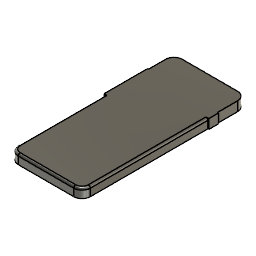
case (Autodesk Fusion 360 design; units mm, degrees)
Autodesk Fusion 360 part; units mm, degrees
sketch "Sketch1" plane through (0, 0, 0) normal (0, 0, 1) x (1, 0, 0)
  line L0 (28.485, 84.19) -> (0, 84.19)
  line L1 (36.985, 0) -> (36.985, 75.69)
  line L2 (0, 0) -> (0, 84.19) construction
  line L3 (0, 0) -> (36.985, 0) construction
  arc A0 (36.985, 75.69) -> (28.485, 84.19) centre (28.485, 75.69) ccw
  line L4 (-28.485, 84.19) -> (0, 84.19)
  arc A1 (-28.485, 84.19) -> (-36.985, 75.69) centre (-28.485, 75.69) ccw
  line L5 (-36.985, 0) -> (-36.985, 75.69)
  line L6 (36.985, 0) -> (36.985, -75.69)
  arc A2 (28.485, -84.19) -> (36.985, -75.69) centre (28.485, -75.69) ccw
  line L7 (28.485, -84.19) -> (0, -84.19)
  line L8 (-28.485, -84.19) -> (0, -84.19)
  arc A3 (-36.985, -75.69) -> (-28.485, -84.19) centre (-28.485, -75.69) ccw
  line L9 (-36.985, 0) -> (-36.985, -75.69)
  line L10 (-36.985, 58.3417) -> (-37.985, 58.3417)
  line L11 (-37.985, 58.3417) -> (-37.985, 38.3417)
  line L12 (-37.985, 38.3417) -> (-36.985, 38.3417)
  line L13 (-36.985, 38.3417) -> (-36.985, 58.3417)
  line L14 (-37.985, 38.3417) -> (-36.985, 38.3417)
  line L15 (-36.985, 38.3417) -> (-36.985, 13.3417)
  line L16 (-36.985, 13.3417) -> (-37.985, 13.3417)
  line L17 (-37.985, 13.3417) -> (-37.985, 38.3417)
  line L18 (36.985, 55.0141) -> (37.985, 55.0141)
  line L19 (37.985, 55.0141) -> (37.985, 45.0141)
  line L20 (37.985, 45.0141) -> (36.985, 45.0141)
  line L21 (36.985, 45.0141) -> (36.985, 55.0141)
  dimension "d3" = 8.5
  dimension "d4" = 1
  dimension "d5" = 20
  dimension "d6" = 25
  dimension "d7" = 1
  dimension "d8" = 10
  constraint horizontal L0
  constraint coincident L2.start L3.start
  constraint tangent L0 A0
  constraint tangent L1 A0
  constraint symmetric L0.end L2 L4.end
  constraint symmetric L2 L1.start L5.start
  constraint symmetric L2 L0.start L4.start
  constraint symmetric L2 L1.end A1.end
  constraint symmetric L2 A0 A1
  constraint symmetric L0.end L3 L7.end
  constraint symmetric L1.start L3 L6.start
  constraint symmetric L3 L0.start A2.start
  constraint symmetric L3 L1.end L6.end
  constraint symmetric L3 A0 A2
  constraint symmetric L3 L4.start L8.start
  constraint symmetric L3 L0.end L7.end
  constraint symmetric L3 A1.end A3.start
  constraint symmetric L3 A1 A3
  constraint symmetric L3 L5.start L9.start
  constraint horizontal L10
  constraint vertical L11
  constraint horizontal L12
  constraint vertical L13
  constraint coincident L5 L10.start
  constraint horizontal L14
  constraint vertical L15
  constraint horizontal L16
  constraint vertical L17
  constraint horizontal L18
  constraint vertical L19
  constraint horizontal L20
  constraint vertical L21
  constraint coincident L1 L18.start
  measures "d3" radius of A0
  measures "d4" distance of L10.start L10.end
  measures "d5" distance of L10.start L12.end
  measures "d6" distance of L11.end L16.end
  measures "d7" distance of L18.start L18.end
  measures "d8" distance of L18.start L20.end
extrude "Extrude1" add sketch "Sketch1" along normal blind 9.69
fillet "Fillet1" radius 2 5 edges at (-36.985, -31.1741, 9.69) (-34.4954, -81.7004, 9.69) (0, -84.19, 9.69) (34.4954, -81.7004, 9.69) (36.985, -15.3379, 9.69)
